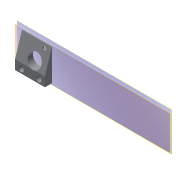
# Autodesk Inventor part: BallCasterMountTemp
Saved by Autodesk Inventor 2018 (Build 220112000, 112)
## iProperties
Created: 2019-02-16
Part Number: BallCasterMountTemp
Material: Generic
Document SubType Name: Modeling
Designer: ball
Density: 1 g/cm^3
Appearance: Default
Author: ball
Autodesk Inventor part; units mm, degrees
ref_plane "Work Plane1" through (0, -45.5, -2.5) normal (0, 0, -1) x (-1, 0, 0)
ref_plane "Work Plane2" through (0, 0, 0) normal (0, 0, 1) x (1, 0, 0)
sketch "Sketch2" plane through (0, 0, 0) normal (0, 0, 1) x (1, 0, 0)
  line L0 (-191.9993, -42.9912) -> (0.0007, -42.9846) construction
  line L1 (-192.0007, 0.0088) -> (0, 0.0154) construction
  line L2 (-192.0007, 0.0088) -> (-191.9993, -42.9912) construction
  circle A0 centre (-168, -21.4904) radius 7.975 construction
  line L3 (-192.0007, 0.0088) -> (-151.3607, 0.0088)
  line L4 (-151.3607, 0.0088) -> (-151.3607, -42.9898)
  line L5 (-151.3607, -42.9898) -> (-192.0007, -42.9898)
  line L6 (-192.0007, -42.9898) -> (-192.0007, 0.0088)
  circle A1 centre (-168, -21.4904) radius 9.2075
  circle A2 centre (-160, -5.5) radius 2 construction
  circle A3 centre (-160, -37.5) radius 2 construction
  circle A4 centre (-160, -5.5) radius 2.1844
  circle A5 centre (-160, -37.5) radius 2.1844
  circle A6 centre (-184, -37.5) radius 2 construction
  circle A7 centre (-184, -37.5) radius 2.1844
  point P0 (0, 0)
  dimension "d0" = 40.64
  dimension "d1" = 18.415
  dimension "d5" = 4.3688
  dimension "d6" = 4.3688
  dimension "d9" = 4.3688
  constraints: 8 end point, 7 centre point, 4 coincident, 2 parallel, 1 horizontal, 1 perpendicular, 1 point on line, 6 other
  measures "d0" distance of L4.end L5.end
  measures "d1" diameter of A1
  measures "d5" diameter of A4
  measures "d6" diameter of A5
  measures "d9" diameter of A7
ref_plane "Work Plane3" through (-192, -45.5, 9.5) normal (0, 0, 1) x (1, 0, 0)
ref_plane "Work Plane4" through (-192, -45.5, 9.5) normal (0, 0, 1) x (1, 0, 0)
ref_plane "Work Plane5" through (-192, 0, 9.5) normal (0, 0, 1) x (1, 0, 0)
extrude "Extrusion3" add sketch "Sketch2" along normal up to surface (9.5 mm away)
sketch "Sketch3" plane through (-192.0007, 0.0088, 9.5) normal (0, 0, 1) x (1, 0, 0)
  circle A0 centre (8.0007, -37.5088) radius 2.1844 projected
  circle A1 centre (32.0007, -37.5088) radius 2.1844 projected
  circle A2 centre (32.0007, -5.5088) radius 2.1844 projected
  point P0 (192.0007, -0.0088)
  constraints: 3 coincident
hole "Hole1" at (-184, -37.5, 9.5) at (-160, -37.5, 9.5) at (-160, -5.5, 9.5) direction (0, 0, -1) diameter 4.3688 end through all counterbore diameter 7.62 counterbore depth 6.985
sketch "Sketch6" plane through (-192.0007, -42.9898, 0) normal (-1, 0, 0) x (0, 0, 1)
  line L0 (4.3851, 29.7217) -> (2.7047, 35.051) construction
  line L1 (0, 42.9986) -> (0, 0) projected
  line L2 (0, 42.9986) -> (9.5, 12.8685)
  line L3 (9.5, 42.9986) -> (9.5, 0) projected
  line L4 (0, 42.9986) -> (31.5923, 42.9986) construction
  line L5 (9.5, 12.8685) -> (9.5, 42.9986)
  line L6 (0, 42.9986) -> (9.5, 42.9986) projected
  line L7 (9.5, 42.9986) -> (0, 42.9986)
  point P0 (0, 42.9898)
  dimension "d23" = 72.5
  constraints: 8 end point, 1 collinear, 1 equal length, 1 horizontal, 1 point on line, 1 vertical
  measures "d23" angle of L2 L4
extrude "Extrusion5" cut sketch "Sketch6" against normal through all
body "Solid3"
